Autodesk Fusion 360 part; units mm, degrees
note: some values were not read from the file. Chosen so that the rebuilt part matches the saved one: which bodies a step acts on.
(part 2 of 5)
sketch "スケッチ1 (6)" plane through (0, 0, 0) normal (0, 0, 1) x (1, 0, 0) in component "Stage1_Planet_Gear_C"
  line L0 (-14.59, -15.7128) -> (-14.4842, -14.6573)
  line L1 (-14.4842, -14.6573) -> (-14.5916, -13.8725)
  line L2 (-14.5916, -13.8725) -> (-14.8686, -13.0785)
  line L3 (-14.8686, -13.0785) -> (-15.2722, -12.2874)
  line L4 (-15.2722, -12.2874) -> (-16.2278, -12.2874)
  line L5 (-16.2278, -12.2874) -> (-16.6314, -13.0785)
  line L6 (-16.6314, -13.0785) -> (-16.9084, -13.8725)
  line L7 (-16.9084, -13.8725) -> (-17.0158, -14.6573)
  line L8 (-17.0158, -14.6573) -> (-16.91, -15.7128)
  line L9 (-16.91, -15.7128) -> (-17.7687, -15.8314)
  line L10 (-17.7687, -15.8314) -> (-18.6161, -16.0137)
  line L11 (-18.6161, -16.0137) -> (-18.8777, -14.9856)
  line L12 (-18.8777, -14.9856) -> (-19.2471, -14.2849)
  line L13 (-19.2471, -14.2849) -> (-19.7789, -13.6335)
  line L14 (-19.7789, -13.6335) -> (-20.4287, -13.0281)
  line L15 (-20.4287, -13.0281) -> (-21.3267, -13.355)
  line L16 (-21.3267, -13.355) -> (-21.4354, -14.2364)
  line L17 (-21.4354, -14.2364) -> (-21.4241, -15.0773)
  line L18 (-21.4241, -15.0773) -> (-21.2566, -15.8514)
  line L19 (-21.2566, -15.8514) -> (-20.7962, -16.8071)
  line L20 (-20.7962, -16.8071) -> (-21.5625, -17.2123)
  line L21 (-21.5625, -17.2123) -> (-22.2965, -17.6734)
  line L22 (-22.2965, -17.6734) -> (-22.8939, -16.7967)
  line L23 (-22.8939, -16.7967) -> (-23.4807, -16.2646)
  line L24 (-23.4807, -16.2646) -> (-24.2032, -15.8344)
  line L25 (-24.2032, -15.8344) -> (-25.0209, -15.4878)
  line L26 (-25.0209, -15.4878) -> (-25.753, -16.1021)
  line L27 (-25.753, -16.1021) -> (-25.5536, -16.9675)
  line L28 (-25.5536, -16.9675) -> (-25.2554, -17.7538)
  line L29 (-25.2554, -17.7538) -> (-24.8333, -18.424)
  line L30 (-24.8333, -18.424) -> (-24.0737, -19.1646)
  line L31 (-24.0737, -19.1646) -> (-24.6553, -19.8074)
  line L32 (-24.6553, -19.8074) -> (-25.1873, -20.4917)
  line L33 (-25.1873, -20.4917) -> (-26.0485, -19.8723)
  line L34 (-26.0485, -19.8723) -> (-26.7819, -19.573)
  line L35 (-26.7819, -19.573) -> (-27.608, -19.4158)
  line L36 (-27.608, -19.4158) -> (-28.4949, -19.3698)
  line L37 (-28.4949, -19.3698) -> (-28.9727, -20.1974)
  line L38 (-28.9727, -20.1974) -> (-28.4894, -20.9425)
  line L39 (-28.4894, -20.9425) -> (-27.9402, -21.5793)
  line L40 (-27.9402, -21.5793) -> (-27.3144, -22.0648)
  line L41 (-27.3144, -22.0648) -> (-26.3473, -22.5009)
  line L42 (-26.3473, -22.5009) -> (-26.6739, -23.3038)
  line L43 (-26.6739, -23.3038) -> (-26.9398, -24.1289)
  line L44 (-26.9398, -24.1289) -> (-27.961, -23.8413)
  line L45 (-27.961, -23.8413) -> (-28.7525, -23.8109)
  line L46 (-28.7525, -23.8109) -> (-29.5825, -23.9458)
  line L47 (-29.5825, -23.9458) -> (-30.4316, -24.2058)
  line L48 (-30.4316, -24.2058) -> (-30.5976, -25.147)
  line L49 (-30.5976, -25.147) -> (-29.8886, -25.6818)
  line L50 (-29.8886, -25.6818) -> (-29.1547, -26.0924)
  line L51 (-29.1547, -26.0924) -> (-28.4006, -26.3345)
  line L52 (-28.4006, -26.3345) -> (-27.3427, -26.4136)
  line L53 (-27.3427, -26.4136) -> (-27.375, -27.2798)
  line L54 (-27.375, -27.2798) -> (-27.3427, -28.146)
  line L55 (-27.3427, -28.146) -> (-28.4006, -28.2251)
  line L56 (-28.4006, -28.2251) -> (-29.1547, -28.4672)
  line L57 (-29.1547, -28.4672) -> (-29.8886, -28.8778)
  line L58 (-29.8886, -28.8778) -> (-30.5976, -29.4126)
  line L59 (-30.5976, -29.4126) -> (-30.4316, -30.3538)
  line L60 (-30.4316, -30.3538) -> (-29.5825, -30.6138)
  line L61 (-29.5825, -30.6138) -> (-28.7525, -30.7487)
  line L62 (-28.7525, -30.7487) -> (-27.961, -30.7183)
  line L63 (-27.961, -30.7183) -> (-26.9398, -30.4307)
  line L64 (-26.9398, -30.4307) -> (-26.6739, -31.2558)
  line L65 (-26.6739, -31.2558) -> (-26.3473, -32.0587)
  line L66 (-26.3473, -32.0587) -> (-27.3144, -32.4948)
  line L67 (-27.3144, -32.4948) -> (-27.9402, -32.9803)
  line L68 (-27.9402, -32.9803) -> (-28.4894, -33.6171)
  line L69 (-28.4894, -33.6171) -> (-28.9727, -34.3622)
  line L70 (-28.9727, -34.3622) -> (-28.4949, -35.1898)
  line L71 (-28.4949, -35.1898) -> (-27.608, -35.1438)
  line L72 (-27.608, -35.1438) -> (-26.7819, -34.9866)
  line L73 (-26.7819, -34.9866) -> (-26.0485, -34.6873)
  line L74 (-26.0485, -34.6873) -> (-25.1873, -34.0679)
  line L75 (-25.1873, -34.0679) -> (-24.6553, -34.7522)
  line L76 (-24.6553, -34.7522) -> (-24.0737, -35.395)
  line L77 (-24.0737, -35.395) -> (-24.8333, -36.1356)
  line L78 (-24.8333, -36.1356) -> (-25.2554, -36.8058)
  line L79 (-25.2554, -36.8058) -> (-25.5536, -37.5921)
  line L80 (-25.5536, -37.5921) -> (-25.753, -38.4575)
  line L81 (-25.753, -38.4575) -> (-25.0209, -39.0718)
  line L82 (-25.0209, -39.0718) -> (-24.2032, -38.7252)
  line L83 (-24.2032, -38.7252) -> (-23.4807, -38.295)
  line L84 (-23.4807, -38.295) -> (-22.8939, -37.7629)
  line L85 (-22.8939, -37.7629) -> (-22.2965, -36.8862)
  line L86 (-22.2965, -36.8862) -> (-21.5625, -37.3473)
  line L87 (-21.5625, -37.3473) -> (-20.7962, -37.7525)
  line L88 (-20.7962, -37.7525) -> (-21.2566, -38.7082)
  line L89 (-21.2566, -38.7082) -> (-21.4241, -39.4823)
  line L90 (-21.4241, -39.4823) -> (-21.4354, -40.3232)
  line L91 (-21.4354, -40.3232) -> (-21.3267, -41.2046)
  line L92 (-21.3267, -41.2046) -> (-20.4287, -41.5315)
  line L93 (-20.4287, -41.5315) -> (-19.7789, -40.9261)
  line L94 (-19.7789, -40.9261) -> (-19.2471, -40.2747)
  line L95 (-19.2471, -40.2747) -> (-18.8777, -39.574)
  line L96 (-18.8777, -39.574) -> (-18.6161, -38.5459)
  line L97 (-18.6161, -38.5459) -> (-17.7687, -38.7282)
  line L98 (-17.7687, -38.7282) -> (-16.91, -38.8468)
  line L99 (-16.91, -38.8468) -> (-17.0158, -39.9023)
  line L100 (-17.0158, -39.9023) -> (-16.9084, -40.6871)
  line L101 (-16.9084, -40.6871) -> (-16.6314, -41.4811)
  line L102 (-16.6314, -41.4811) -> (-16.2278, -42.2722)
  line L103 (-16.2278, -42.2722) -> (-15.2722, -42.2722)
  line L104 (-15.2722, -42.2722) -> (-14.8686, -41.4811)
  line L105 (-14.8686, -41.4811) -> (-14.5916, -40.6871)
  line L106 (-14.5916, -40.6871) -> (-14.4842, -39.9023)
  line L107 (-14.4842, -39.9023) -> (-14.59, -38.8468)
  line L108 (-14.59, -38.8468) -> (-13.7313, -38.7282)
  line L109 (-13.7313, -38.7282) -> (-12.8839, -38.5459)
  line L110 (-12.8839, -38.5459) -> (-12.6223, -39.574)
  line L111 (-12.6223, -39.574) -> (-12.2529, -40.2747)
  line L112 (-12.2529, -40.2747) -> (-11.7211, -40.9261)
  line L113 (-11.7211, -40.9261) -> (-11.0713, -41.5315)
  line L114 (-11.0713, -41.5315) -> (-10.1733, -41.2046)
  line L115 (-10.1733, -41.2046) -> (-10.0646, -40.3232)
  line L116 (-10.0646, -40.3232) -> (-10.0759, -39.4823)
  line L117 (-10.0759, -39.4823) -> (-10.2434, -38.7082)
  line L118 (-10.2434, -38.7082) -> (-10.7038, -37.7525)
  line L119 (-10.7038, -37.7525) -> (-9.9375, -37.3473)
  line L120 (-9.9375, -37.3473) -> (-9.2035, -36.8862)
  line L121 (-9.2035, -36.8862) -> (-8.6061, -37.7629)
  line L122 (-8.6061, -37.7629) -> (-8.0193, -38.295)
  line L123 (-8.0193, -38.295) -> (-7.2968, -38.7252)
  line L124 (-7.2968, -38.7252) -> (-6.4791, -39.0718)
  line L125 (-6.4791, -39.0718) -> (-5.747, -38.4575)
  line L126 (-5.747, -38.4575) -> (-5.9464, -37.5921)
  line L127 (-5.9464, -37.5921) -> (-6.2446, -36.8058)
  line L128 (-6.2446, -36.8058) -> (-6.6667, -36.1356)
  line L129 (-6.6667, -36.1356) -> (-7.4263, -35.395)
  line L130 (-7.4263, -35.395) -> (-6.8447, -34.7522)
  line L131 (-6.8447, -34.7522) -> (-6.3127, -34.0679)
  line L132 (-6.3127, -34.0679) -> (-5.4515, -34.6873)
  line L133 (-5.4515, -34.6873) -> (-4.7181, -34.9866)
  line L134 (-4.7181, -34.9866) -> (-3.892, -35.1438)
  line L135 (-3.892, -35.1438) -> (-3.0051, -35.1898)
  line L136 (-3.0051, -35.1898) -> (-2.5273, -34.3622)
  line L137 (-2.5273, -34.3622) -> (-3.0106, -33.6171)
  line L138 (-3.0106, -33.6171) -> (-3.5598, -32.9803)
  line L139 (-3.5598, -32.9803) -> (-4.1856, -32.4948)
  line L140 (-4.1856, -32.4948) -> (-5.1527, -32.0587)
  line L141 (-5.1527, -32.0587) -> (-4.8261, -31.2558)
  line L142 (-4.8261, -31.2558) -> (-4.5602, -30.4307)
  line L143 (-4.5602, -30.4307) -> (-3.539, -30.7183)
  line L144 (-3.539, -30.7183) -> (-2.7475, -30.7487)
  line L145 (-2.7475, -30.7487) -> (-1.9175, -30.6138)
  line L146 (-1.9175, -30.6138) -> (-1.0684, -30.3538)
  line L147 (-1.0684, -30.3538) -> (-0.9024, -29.4126)
  line L148 (-0.9024, -29.4126) -> (-1.6114, -28.8778)
  line L149 (-1.6114, -28.8778) -> (-2.3453, -28.4672)
  line L150 (-2.3453, -28.4672) -> (-3.0994, -28.2251)
  line L151 (-3.0994, -28.2251) -> (-4.1573, -28.146)
  line L152 (-4.1573, -28.146) -> (-4.125, -27.2798)
  line L153 (-4.125, -27.2798) -> (-4.1573, -26.4136)
  line L154 (-4.1573, -26.4136) -> (-3.0994, -26.3345)
  line L155 (-3.0994, -26.3345) -> (-2.3453, -26.0924)
  line L156 (-2.3453, -26.0924) -> (-1.6114, -25.6818)
  line L157 (-1.6114, -25.6818) -> (-0.9024, -25.147)
  line L158 (-0.9024, -25.147) -> (-1.0684, -24.2058)
  line L159 (-1.0684, -24.2058) -> (-1.9175, -23.9458)
  line L160 (-1.9175, -23.9458) -> (-2.7475, -23.8109)
  line L161 (-2.7475, -23.8109) -> (-3.539, -23.8413)
  line L162 (-3.539, -23.8413) -> (-4.5602, -24.1289)
  line L163 (-4.5602, -24.1289) -> (-4.8261, -23.3038)
  line L164 (-4.8261, -23.3038) -> (-5.1527, -22.5009)
  line L165 (-5.1527, -22.5009) -> (-4.1856, -22.0648)
  line L166 (-4.1856, -22.0648) -> (-3.5598, -21.5793)
  line L167 (-3.5598, -21.5793) -> (-3.0106, -20.9425)
  line L168 (-3.0106, -20.9425) -> (-2.5273, -20.1974)
  line L169 (-2.5273, -20.1974) -> (-3.0051, -19.3698)
  line L170 (-3.0051, -19.3698) -> (-3.892, -19.4158)
  line L171 (-3.892, -19.4158) -> (-4.7181, -19.573)
  line L172 (-4.7181, -19.573) -> (-5.4515, -19.8723)
  line L173 (-5.4515, -19.8723) -> (-6.3127, -20.4917)
  line L174 (-6.3127, -20.4917) -> (-6.8447, -19.8074)
  line L175 (-6.8447, -19.8074) -> (-7.4263, -19.1646)
  line L176 (-7.4263, -19.1646) -> (-6.6667, -18.424)
  line L177 (-6.6667, -18.424) -> (-6.2446, -17.7538)
  line L178 (-6.2446, -17.7538) -> (-5.9464, -16.9675)
  line L179 (-5.9464, -16.9675) -> (-5.747, -16.1021)
  line L180 (-5.747, -16.1021) -> (-6.4791, -15.4878)
  line L181 (-6.4791, -15.4878) -> (-7.2968, -15.8344)
  line L182 (-7.2968, -15.8344) -> (-8.0193, -16.2646)
  line L183 (-8.0193, -16.2646) -> (-8.6061, -16.7967)
  line L184 (-8.6061, -16.7967) -> (-9.2035, -17.6734)
  line L185 (-9.2035, -17.6734) -> (-9.9375, -17.2123)
  line L186 (-9.9375, -17.2123) -> (-10.7038, -16.8071)
  line L187 (-10.7038, -16.8071) -> (-10.2434, -15.8514)
  line L188 (-10.2434, -15.8514) -> (-10.0759, -15.0773)
  line L189 (-10.0759, -15.0773) -> (-10.0646, -14.2364)
  line L190 (-10.0646, -14.2364) -> (-10.1733, -13.355)
  line L191 (-10.1733, -13.355) -> (-11.0713, -13.0281)
  line L192 (-11.0713, -13.0281) -> (-11.7211, -13.6335)
  line L193 (-11.7211, -13.6335) -> (-12.2529, -14.2849)
  line L194 (-12.2529, -14.2849) -> (-12.6223, -14.9856)
  line L195 (-12.6223, -14.9856) -> (-12.8839, -16.0137)
  line L196 (-12.8839, -16.0137) -> (-13.7313, -15.8314)
  line L197 (-13.7313, -15.8314) -> (-14.59, -15.7128)
extrude "Stage1_Planet_C_Extrude" add sketch "スケッチ1 (6)" along normal blind 12 from surface at 34 separate body makes body 6 in component "Stage1_Planet_Gear_C"
sketch "スケッチ2 (6)" plane through (0, 0, 0) normal (0, 0, 1) x (1, 0, 0) in component "Stage1_Planet_Gear_C"
  circle A0 centre (-15.75, -27.2798) radius 8
extrude "Stage1_Planet_C_Hub_Lower_Extrude" add sketch "スケッチ2 (6)" along normal blind 3.5 from surface at 30.5 bodies 6 in component "Stage1_Planet_Gear_C"
sketch "スケッチ3 (6)" plane through (0, 0, 0) normal (0, 0, 1) x (1, 0, 0) in component "Stage1_Planet_Gear_C"
  circle A0 centre (-15.75, -27.2798) radius 8
extrude "Stage1_Planet_C_Hub_Upper_Extrude" add sketch "スケッチ3 (6)" along normal blind 3.5 from surface at 46 bodies 6 in component "Stage1_Planet_Gear_C"
sketch "スケッチ4 (6)" plane through (0, 0, 0) normal (0, 0, 1) x (1, 0, 0) in component "Stage1_Planet_Gear_C"
  circle A0 centre (-15.75, -27.2798) radius 4.3
extrude "Stage1_Planet_C_Bore_Cut" cut sketch "スケッチ4 (6)" along normal blind 22 from surface at 29 bodies 6 in component "Stage1_Planet_Gear_C"
sketch "スケッチ1 (7)" plane through (0, 0, 0) normal (0, 0, 1) x (1, 0, 0) in component "Stage1_Internal_Ring_Gear"
  circle A0 centre (0, 0) radius 58
extrude "Stage1_Ring_Extrude" add sketch "スケッチ1 (7)" along normal blind 12 from surface at 34 separate body makes body 7 in component "Stage1_Internal_Ring_Gear"
sketch "スケッチ2 (7)" plane through (0, 0, 0) normal (0, 0, 1) x (1, 0, 0) in component "Stage1_Internal_Ring_Gear"
  circle A0 centre (0, 0) radius 65.5
extrude "Stage1_Ring_Flange_Extrude" add sketch "スケッチ2 (7)" along normal blind 7 from surface at 36.5 bodies 7 in component "Stage1_Internal_Ring_Gear"
sketch "スケッチ3 (7)" plane through (0, 0, 0) normal (0, 0, 1) x (1, 0, 0) in component "Stage1_Internal_Ring_Gear"
  line L0 (46.8321, -2.0047) -> (45.171, -1.2223)
  line L1 (45.171, -1.2223) -> (43.495, -0.6584)
  line L2 (43.495, -0.6584) -> (43.495, 0.6584)
  line L3 (43.495, 0.6584) -> (45.171, 1.2223)
  line L4 (45.171, 1.2223) -> (46.8321, 2.0047)
  line L5 (46.8321, 2.0047) -> (46.8108, 2.4532)
  line L6 (46.8108, 2.4532) -> (46.7851, 2.9016)
  line L7 (46.7851, 2.9016) -> (45.0513, 3.506)
  line L8 (45.0513, 3.506) -> (43.3256, 3.8917)
  line L9 (43.3256, 3.8917) -> (43.1879, 5.2013)
  line L10 (43.1879, 5.2013) -> (44.7957, 5.9373)
  line L11 (44.7957, 5.9373) -> (46.366, 6.889)
  line L12 (46.366, 6.889) -> (46.2979, 7.3329)
  line L13 (46.2979, 7.3329) -> (46.2255, 7.7761)
  line L14 (46.2255, 7.7761) -> (44.438, 8.196)
  line L15 (44.438, 8.196) -> (42.6814, 8.3991)
  line L16 (42.6814, 8.3991) -> (42.4077, 9.6871)
  line L17 (42.4077, 9.6871) -> (43.9297, 10.5872)
  line L18 (43.9297, 10.5872) -> (45.3919, 11.6978)
  line L19 (45.3919, 11.6978) -> (45.2778, 12.1321)
  line L20 (45.2778, 12.1321) -> (45.1595, 12.5653)
  line L21 (45.1595, 12.5653) -> (43.3379, 12.7961)
  line L22 (43.3379, 12.7961) -> (41.5697, 12.8145)
  line L23 (41.5697, 12.8145) -> (41.1628, 14.0669)
  line L24 (41.1628, 14.0669) -> (42.5824, 15.1211)
  line L25 (42.5824, 15.1211) -> (43.9205, 16.3785)
  line L26 (43.9205, 16.3785) -> (43.7616, 16.7985)
  line L27 (43.7616, 16.7985) -> (43.5986, 17.217)
  line L28 (43.5986, 17.217) -> (41.7629, 17.256)
  line L29 (41.7629, 17.256) -> (40.0025, 17.0895)
  line L30 (40.0025, 17.0895) -> (39.4669, 18.2925)
  line L31 (39.4669, 18.2925) -> (40.7686, 19.4893)
  line L32 (40.7686, 19.4893) -> (41.9679, 20.8797)
  line L33 (41.9679, 20.8797) -> (41.7659, 21.2808)
  line L34 (41.7659, 21.2808) -> (41.5601, 21.6799)
  line L35 (41.5601, 21.6799) -> (39.7304, 21.5269)
  line L36 (39.7304, 21.5269) -> (37.997, 21.1773)
  line L37 (37.997, 21.1773) -> (37.3386, 22.3177)
  line L38 (37.3386, 22.3177) -> (38.508, 23.644)
  line L39 (38.508, 23.644) -> (39.5555, 25.1522)
  line L40 (39.5555, 25.1522) -> (39.3127, 25.53)
  line L41 (39.3127, 25.53) -> (39.0663, 25.9054)
  line L42 (39.0663, 25.9054) -> (37.2625, 25.5619)
  line L43 (37.2625, 25.5619) -> (35.5752, 25.0331)
  line L44 (35.5752, 25.0331) -> (34.8012, 26.0984)
  line L45 (34.8012, 26.0984) -> (35.8256, 27.5397)
  line L46 (35.8256, 27.5397) -> (36.7096, 29.1491)
  line L47 (36.7096, 29.1491) -> (36.4287, 29.4994)
  line L48 (36.4287, 29.4994) -> (36.1444, 29.847)
  line L49 (36.1444, 29.847) -> (34.3865, 29.3169)
  line L50 (34.3865, 29.3169) -> (32.7636, 28.6146)
  line L51 (32.7636, 28.6146) -> (31.8825, 29.5931)
  line L52 (31.8825, 29.5931) -> (32.7507, 31.1336)
  line L53 (32.7507, 31.1336) -> (33.4616, 32.8266)
  line L54 (33.4616, 32.8266) -> (33.1456, 33.1456)
  line L55 (33.1456, 33.1456) -> (32.8266, 33.4616)
  line L56 (32.8266, 33.4616) -> (31.1336, 32.7507)
  line L57 (31.1336, 32.7507) -> (29.5931, 31.8825)
  line L58 (29.5931, 31.8825) -> (28.6146, 32.7636)
  line L59 (28.6146, 32.7636) -> (29.3169, 34.3865)
  line L60 (29.3169, 34.3865) -> (29.847, 36.1444)
  line L61 (29.847, 36.1444) -> (29.4994, 36.4287)
  line L62 (29.4994, 36.4287) -> (29.1491, 36.7096)
  line L63 (29.1491, 36.7096) -> (27.5397, 35.8256)
  line L64 (27.5397, 35.8256) -> (26.0984, 34.8012)
  line L65 (26.0984, 34.8012) -> (25.0331, 35.5752)
  line L66 (25.0331, 35.5752) -> (25.5619, 37.2625)
  line L67 (25.5619, 37.2625) -> (25.9054, 39.0663)
  line L68 (25.9054, 39.0663) -> (25.53, 39.3127)
  line L69 (25.53, 39.3127) -> (25.1522, 39.5555)
  line L70 (25.1522, 39.5555) -> (23.644, 38.508)
  line L71 (23.644, 38.508) -> (22.3177, 37.3386)
  line L72 (22.3177, 37.3386) -> (21.1773, 37.997)
  line L73 (21.1773, 37.997) -> (21.5269, 39.7304)
  line L74 (21.5269, 39.7304) -> (21.6799, 41.5601)
  line L75 (21.6799, 41.5601) -> (21.2808, 41.7659)
  line L76 (21.2808, 41.7659) -> (20.8797, 41.9679)
  line L77 (20.8797, 41.9679) -> (19.4893, 40.7686)
  line L78 (19.4893, 40.7686) -> (18.2925, 39.4669)
  line L79 (18.2925, 39.4669) -> (17.0895, 40.0025)
  line L80 (17.0895, 40.0025) -> (17.256, 41.7629)
  line L81 (17.256, 41.7629) -> (17.217, 43.5986)
  line L82 (17.217, 43.5986) -> (16.7985, 43.7616)
  line L83 (16.7985, 43.7616) -> (16.3785, 43.9205)
  line L84 (16.3785, 43.9205) -> (15.1211, 42.5824)
  line L85 (15.1211, 42.5824) -> (14.0669, 41.1628)
  line L86 (14.0669, 41.1628) -> (12.8145, 41.5697)
  line L87 (12.8145, 41.5697) -> (12.7961, 43.3379)
  line L88 (12.7961, 43.3379) -> (12.5653, 45.1595)
  line L89 (12.5653, 45.1595) -> (12.1321, 45.2778)
  line L90 (12.1321, 45.2778) -> (11.6978, 45.3919)
  line L91 (11.6978, 45.3919) -> (10.5872, 43.9297)
  line L92 (10.5872, 43.9297) -> (9.6871, 42.4077)
  line L93 (9.6871, 42.4077) -> (8.3991, 42.6814)
  line L94 (8.3991, 42.6814) -> (8.196, 44.438)
  line L95 (8.196, 44.438) -> (7.7761, 46.2255)
  line L96 (7.7761, 46.2255) -> (7.3329, 46.2979)
  line L97 (7.3329, 46.2979) -> (6.889, 46.366)
  line L98 (6.889, 46.366) -> (5.9373, 44.7957)
  line L99 (5.9373, 44.7957) -> (5.2013, 43.1879)
  line L100 (5.2013, 43.1879) -> (3.8917, 43.3256)
  line L101 (3.8917, 43.3256) -> (3.506, 45.0513)
  line L102 (3.506, 45.0513) -> (2.9016, 46.7851)
  line L103 (2.9016, 46.7851) -> (2.4532, 46.8108)
  line L104 (2.4532, 46.8108) -> (2.0047, 46.8321)
  line L105 (2.0047, 46.8321) -> (1.2223, 45.171)
  line L106 (1.2223, 45.171) -> (0.6584, 43.495)
  line L107 (0.6584, 43.495) -> (-0.6584, 43.495)
  line L108 (-0.6584, 43.495) -> (-1.2223, 45.171)
  line L109 (-1.2223, 45.171) -> (-2.0047, 46.8321)
  line L110 (-2.0047, 46.8321) -> (-2.4532, 46.8108)
  line L111 (-2.4532, 46.8108) -> (-2.9016, 46.7851)
  line L112 (-2.9016, 46.7851) -> (-3.506, 45.0513)
  line L113 (-3.506, 45.0513) -> (-3.8917, 43.3256)
  line L114 (-3.8917, 43.3256) -> (-5.2013, 43.1879)
  line L115 (-5.2013, 43.1879) -> (-5.9373, 44.7957)
  line L116 (-5.9373, 44.7957) -> (-6.889, 46.366)
  line L117 (-6.889, 46.366) -> (-7.3329, 46.2979)
  line L118 (-7.3329, 46.2979) -> (-7.7761, 46.2255)
  line L119 (-7.7761, 46.2255) -> (-8.196, 44.438)
  line L120 (-8.196, 44.438) -> (-8.3991, 42.6814)
  line L121 (-8.3991, 42.6814) -> (-9.6871, 42.4077)
  line L122 (-9.6871, 42.4077) -> (-10.5872, 43.9297)
  line L123 (-10.5872, 43.9297) -> (-11.6978, 45.3919)
  line L124 (-11.6978, 45.3919) -> (-12.1321, 45.2778)
  line L125 (-12.1321, 45.2778) -> (-12.5653, 45.1595)
  line L126 (-12.5653, 45.1595) -> (-12.7961, 43.3379)
  line L127 (-12.7961, 43.3379) -> (-12.8145, 41.5697)
  line L128 (-12.8145, 41.5697) -> (-14.0669, 41.1628)
  line L129 (-14.0669, 41.1628) -> (-15.1211, 42.5824)
  line L130 (-15.1211, 42.5824) -> (-16.3785, 43.9205)
  line L131 (-16.3785, 43.9205) -> (-16.7985, 43.7616)
  line L132 (-16.7985, 43.7616) -> (-17.217, 43.5986)
  line L133 (-17.217, 43.5986) -> (-17.256, 41.7629)
  line L134 (-17.256, 41.7629) -> (-17.0895, 40.0025)
  line L135 (-17.0895, 40.0025) -> (-18.2925, 39.4669)
  line L136 (-18.2925, 39.4669) -> (-19.4893, 40.7686)
  line L137 (-19.4893, 40.7686) -> (-20.8797, 41.9679)
  line L138 (-20.8797, 41.9679) -> (-21.2808, 41.7659)
  line L139 (-21.2808, 41.7659) -> (-21.6799, 41.5601)
  line L140 (-21.6799, 41.5601) -> (-21.5269, 39.7304)
  line L141 (-21.5269, 39.7304) -> (-21.1773, 37.997)
  line L142 (-21.1773, 37.997) -> (-22.3177, 37.3386)
  line L143 (-22.3177, 37.3386) -> (-23.644, 38.508)
  line L144 (-23.644, 38.508) -> (-25.1522, 39.5555)
  line L145 (-25.1522, 39.5555) -> (-25.53, 39.3127)
  line L146 (-25.53, 39.3127) -> (-25.9054, 39.0663)
  line L147 (-25.9054, 39.0663) -> (-25.5619, 37.2625)
  line L148 (-25.5619, 37.2625) -> (-25.0331, 35.5752)
  line L149 (-25.0331, 35.5752) -> (-26.0984, 34.8012)
  line L150 (-26.0984, 34.8012) -> (-27.5397, 35.8256)
  line L151 (-27.5397, 35.8256) -> (-29.1491, 36.7096)
  line L152 (-29.1491, 36.7096) -> (-29.4994, 36.4287)
  line L153 (-29.4994, 36.4287) -> (-29.847, 36.1444)
  line L154 (-29.847, 36.1444) -> (-29.3169, 34.3865)
  line L155 (-29.3169, 34.3865) -> (-28.6146, 32.7636)
  line L156 (-28.6146, 32.7636) -> (-29.5931, 31.8825)
  line L157 (-29.5931, 31.8825) -> (-31.1336, 32.7507)
  line L158 (-31.1336, 32.7507) -> (-32.8266, 33.4616)
  line L159 (-32.8266, 33.4616) -> (-33.1456, 33.1456)
  line L160 (-33.1456, 33.1456) -> (-33.4616, 32.8266)
  line L161 (-33.4616, 32.8266) -> (-32.7507, 31.1336)
  line L162 (-32.7507, 31.1336) -> (-31.8825, 29.5931)
  line L163 (-31.8825, 29.5931) -> (-32.7636, 28.6146)
  line L164 (-32.7636, 28.6146) -> (-34.3865, 29.3169)
  line L165 (-34.3865, 29.3169) -> (-36.1444, 29.847)
  line L166 (-36.1444, 29.847) -> (-36.4287, 29.4994)
  line L167 (-36.4287, 29.4994) -> (-36.7096, 29.1491)
  line L168 (-36.7096, 29.1491) -> (-35.8256, 27.5397)
  line L169 (-35.8256, 27.5397) -> (-34.8012, 26.0984)
  line L170 (-34.8012, 26.0984) -> (-35.5752, 25.0331)
  line L171 (-35.5752, 25.0331) -> (-37.2625, 25.5619)
  line L172 (-37.2625, 25.5619) -> (-39.0663, 25.9054)
  line L173 (-39.0663, 25.9054) -> (-39.3127, 25.53)
  line L174 (-39.3127, 25.53) -> (-39.5555, 25.1522)
  line L175 (-39.5555, 25.1522) -> (-38.508, 23.644)
  line L176 (-38.508, 23.644) -> (-37.3386, 22.3177)
  line L177 (-37.3386, 22.3177) -> (-37.997, 21.1773)
  line L178 (-37.997, 21.1773) -> (-39.7304, 21.5269)
  line L179 (-39.7304, 21.5269) -> (-41.5601, 21.6799)
  line L180 (-41.5601, 21.6799) -> (-41.7659, 21.2808)
  line L181 (-41.7659, 21.2808) -> (-41.9679, 20.8797)
  line L182 (-41.9679, 20.8797) -> (-40.7686, 19.4893)
  line L183 (-40.7686, 19.4893) -> (-39.4669, 18.2925)
  line L184 (-39.4669, 18.2925) -> (-40.0025, 17.0895)
  line L185 (-40.0025, 17.0895) -> (-41.7629, 17.256)
  line L186 (-41.7629, 17.256) -> (-43.5986, 17.217)
  line L187 (-43.5986, 17.217) -> (-43.7616, 16.7985)
  line L188 (-43.7616, 16.7985) -> (-43.9205, 16.3785)
  line L189 (-43.9205, 16.3785) -> (-42.5824, 15.1211)
  line L190 (-42.5824, 15.1211) -> (-41.1628, 14.0669)
  line L191 (-41.1628, 14.0669) -> (-41.5697, 12.8145)
  line L192 (-41.5697, 12.8145) -> (-43.3379, 12.7961)
  line L193 (-43.3379, 12.7961) -> (-45.1595, 12.5653)
  line L194 (-45.1595, 12.5653) -> (-45.2778, 12.1321)
  line L195 (-45.2778, 12.1321) -> (-45.3919, 11.6978)
  line L196 (-45.3919, 11.6978) -> (-43.9297, 10.5872)
  line L197 (-43.9297, 10.5872) -> (-42.4077, 9.6871)
  line L198 (-42.4077, 9.6871) -> (-42.6814, 8.3991)
  line L199 (-42.6814, 8.3991) -> (-44.438, 8.196)
  line L200 (-44.438, 8.196) -> (-46.2255, 7.7761)
  line L201 (-46.2255, 7.7761) -> (-46.2979, 7.3329)
  line L202 (-46.2979, 7.3329) -> (-46.366, 6.889)
  line L203 (-46.366, 6.889) -> (-44.7957, 5.9373)
  line L204 (-44.7957, 5.9373) -> (-43.1879, 5.2013)
  line L205 (-43.1879, 5.2013) -> (-43.3256, 3.8917)
  line L206 (-43.3256, 3.8917) -> (-45.0513, 3.506)
  line L207 (-45.0513, 3.506) -> (-46.7851, 2.9016)
  line L208 (-46.7851, 2.9016) -> (-46.8108, 2.4532)
  line L209 (-46.8108, 2.4532) -> (-46.8321, 2.0047)
  line L210 (-46.8321, 2.0047) -> (-45.171, 1.2223)
  line L211 (-45.171, 1.2223) -> (-43.495, 0.6584)
  line L212 (-43.495, 0.6584) -> (-43.495, -0.6584)
  line L213 (-43.495, -0.6584) -> (-45.171, -1.2223)
  line L214 (-45.171, -1.2223) -> (-46.8321, -2.0047)
  line L215 (-46.8321, -2.0047) -> (-46.8108, -2.4532)
  line L216 (-46.8108, -2.4532) -> (-46.7851, -2.9016)
  line L217 (-46.7851, -2.9016) -> (-45.0513, -3.506)
  line L218 (-45.0513, -3.506) -> (-43.3256, -3.8917)
  line L219 (-43.3256, -3.8917) -> (-43.1879, -5.2013)
  line L220 (-43.1879, -5.2013) -> (-44.7957, -5.9373)
  line L221 (-44.7957, -5.9373) -> (-46.366, -6.889)
  line L222 (-46.366, -6.889) -> (-46.2979, -7.3329)
  line L223 (-46.2979, -7.3329) -> (-46.2255, -7.7761)
  line L224 (-46.2255, -7.7761) -> (-44.438, -8.196)
  line L225 (-44.438, -8.196) -> (-42.6814, -8.3991)
  line L226 (-42.6814, -8.3991) -> (-42.4077, -9.6871)
  line L227 (-42.4077, -9.6871) -> (-43.9297, -10.5872)
  line L228 (-43.9297, -10.5872) -> (-45.3919, -11.6978)
  line L229 (-45.3919, -11.6978) -> (-45.2778, -12.1321)
  line L230 (-45.2778, -12.1321) -> (-45.1595, -12.5653)
  line L231 (-45.1595, -12.5653) -> (-43.3379, -12.7961)
  line L232 (-43.3379, -12.7961) -> (-41.5697, -12.8145)
  line L233 (-41.5697, -12.8145) -> (-41.1628, -14.0669)
  line L234 (-41.1628, -14.0669) -> (-42.5824, -15.1211)
  line L235 (-42.5824, -15.1211) -> (-43.9205, -16.3785)
  line L236 (-43.9205, -16.3785) -> (-43.7616, -16.7985)
  line L237 (-43.7616, -16.7985) -> (-43.5986, -17.217)
  line L238 (-43.5986, -17.217) -> (-41.7629, -17.256)
  line L239 (-41.7629, -17.256) -> (-40.0025, -17.0895)
  line L240 (-40.0025, -17.0895) -> (-39.4669, -18.2925)
  line L241 (-39.4669, -18.2925) -> (-40.7686, -19.4893)
  line L242 (-40.7686, -19.4893) -> (-41.9679, -20.8797)
  line L243 (-41.9679, -20.8797) -> (-41.7659, -21.2808)
  line L244 (-41.7659, -21.2808) -> (-41.5601, -21.6799)
  line L245 (-41.5601, -21.6799) -> (-39.7304, -21.5269)
  line L246 (-39.7304, -21.5269) -> (-37.997, -21.1773)
  line L247 (-37.997, -21.1773) -> (-37.3386, -22.3177)
  line L248 (-37.3386, -22.3177) -> (-38.508, -23.644)
  line L249 (-38.508, -23.644) -> (-39.5555, -25.1522)
  line L250 (-39.5555, -25.1522) -> (-39.3127, -25.53)
  line L251 (-39.3127, -25.53) -> (-39.0663, -25.9054)
  line L252 (-39.0663, -25.9054) -> (-37.2625, -25.5619)
  line L253 (-37.2625, -25.5619) -> (-35.5752, -25.0331)
  line L254 (-35.5752, -25.0331) -> (-34.8012, -26.0984)
  line L255 (-34.8012, -26.0984) -> (-35.8256, -27.5397)
  line L256 (-35.8256, -27.5397) -> (-36.7096, -29.1491)
  line L257 (-36.7096, -29.1491) -> (-36.4287, -29.4994)
  line L258 (-36.4287, -29.4994) -> (-36.1444, -29.847)
  line L259 (-36.1444, -29.847) -> (-34.3865, -29.3169)
  line L260 (-34.3865, -29.3169) -> (-32.7636, -28.6146)
  line L261 (-32.7636, -28.6146) -> (-31.8825, -29.5931)
  line L262 (-31.8825, -29.5931) -> (-32.7507, -31.1336)
  line L263 (-32.7507, -31.1336) -> (-33.4616, -32.8266)
  line L264 (-33.4616, -32.8266) -> (-33.1456, -33.1456)
  line L265 (-33.1456, -33.1456) -> (-32.8266, -33.4616)
  line L266 (-32.8266, -33.4616) -> (-31.1336, -32.7507)
  line L267 (-31.1336, -32.7507) -> (-29.5931, -31.8825)
  line L268 (-29.5931, -31.8825) -> (-28.6146, -32.7636)
  line L269 (-28.6146, -32.7636) -> (-29.3169, -34.3865)
  line L270 (-29.3169, -34.3865) -> (-29.847, -36.1444)
  line L271 (-29.847, -36.1444) -> (-29.4994, -36.4287)
  line L272 (-29.4994, -36.4287) -> (-29.1491, -36.7096)
  line L273 (-29.1491, -36.7096) -> (-27.5397, -35.8256)
  line L274 (-27.5397, -35.8256) -> (-26.0984, -34.8012)
  line L275 (-26.0984, -34.8012) -> (-25.0331, -35.5752)
  line L276 (-25.0331, -35.5752) -> (-25.5619, -37.2625)
  line L277 (-25.5619, -37.2625) -> (-25.9054, -39.0663)
  line L278 (-25.9054, -39.0663) -> (-25.53, -39.3127)
  line L279 (-25.53, -39.3127) -> (-25.1522, -39.5555)
  line L280 (-25.1522, -39.5555) -> (-23.644, -38.508)
  line L281 (-23.644, -38.508) -> (-22.3177, -37.3386)
  line L282 (-22.3177, -37.3386) -> (-21.1773, -37.997)
  line L283 (-21.1773, -37.997) -> (-21.5269, -39.7304)
  line L284 (-21.5269, -39.7304) -> (-21.6799, -41.5601)
  line L285 (-21.6799, -41.5601) -> (-21.2808, -41.7659)
  line L286 (-21.2808, -41.7659) -> (-20.8797, -41.9679)
  line L287 (-20.8797, -41.9679) -> (-19.4893, -40.7686)
  line L288 (-19.4893, -40.7686) -> (-18.2925, -39.4669)
  line L289 (-18.2925, -39.4669) -> (-17.0895, -40.0025)
  line L290 (-17.0895, -40.0025) -> (-17.256, -41.7629)
  line L291 (-17.256, -41.7629) -> (-17.217, -43.5986)
  line L292 (-17.217, -43.5986) -> (-16.7985, -43.7616)
  line L293 (-16.7985, -43.7616) -> (-16.3785, -43.9205)
  line L294 (-16.3785, -43.9205) -> (-15.1211, -42.5824)
  line L295 (-15.1211, -42.5824) -> (-14.0669, -41.1628)
  line L296 (-14.0669, -41.1628) -> (-12.8145, -41.5697)
  line L297 (-12.8145, -41.5697) -> (-12.7961, -43.3379)
  line L298 (-12.7961, -43.3379) -> (-12.5653, -45.1595)
  line L299 (-12.5653, -45.1595) -> (-12.1321, -45.2778)
  line L300 (-12.1321, -45.2778) -> (-11.6978, -45.3919)
  line L301 (-11.6978, -45.3919) -> (-10.5872, -43.9297)
  line L302 (-10.5872, -43.9297) -> (-9.6871, -42.4077)
  line L303 (-9.6871, -42.4077) -> (-8.3991, -42.6814)
  line L304 (-8.3991, -42.6814) -> (-8.196, -44.438)
  line L305 (-8.196, -44.438) -> (-7.7761, -46.2255)
  line L306 (-7.7761, -46.2255) -> (-7.3329, -46.2979)
  line L307 (-7.3329, -46.2979) -> (-6.889, -46.366)
  line L308 (-6.889, -46.366) -> (-5.9373, -44.7957)
  line L309 (-5.9373, -44.7957) -> (-5.2013, -43.1879)
  line L310 (-5.2013, -43.1879) -> (-3.8917, -43.3256)
  line L311 (-3.8917, -43.3256) -> (-3.506, -45.0513)
  line L312 (-3.506, -45.0513) -> (-2.9016, -46.7851)
  line L313 (-2.9016, -46.7851) -> (-2.4532, -46.8108)
  line L314 (-2.4532, -46.8108) -> (-2.0047, -46.8321)
  line L315 (-2.0047, -46.8321) -> (-1.2223, -45.171)
  line L316 (-1.2223, -45.171) -> (-0.6584, -43.495)
  line L317 (-0.6584, -43.495) -> (0.6584, -43.495)
  line L318 (0.6584, -43.495) -> (1.2223, -45.171)
  line L319 (1.2223, -45.171) -> (2.0047, -46.8321)
  line L320 (2.0047, -46.8321) -> (2.4532, -46.8108)
  line L321 (2.4532, -46.8108) -> (2.9016, -46.7851)
  line L322 (2.9016, -46.7851) -> (3.506, -45.0513)
  line L323 (3.506, -45.0513) -> (3.8917, -43.3256)
  line L324 (3.8917, -43.3256) -> (5.2013, -43.1879)
  line L325 (5.2013, -43.1879) -> (5.9373, -44.7957)
  line L326 (5.9373, -44.7957) -> (6.889, -46.366)
  line L327 (6.889, -46.366) -> (7.3329, -46.2979)
  line L328 (7.3329, -46.2979) -> (7.7761, -46.2255)
  line L329 (7.7761, -46.2255) -> (8.196, -44.438)
  line L330 (8.196, -44.438) -> (8.3991, -42.6814)
  line L331 (8.3991, -42.6814) -> (9.6871, -42.4077)
  line L332 (9.6871, -42.4077) -> (10.5872, -43.9297)
  line L333 (10.5872, -43.9297) -> (11.6978, -45.3919)
  line L334 (11.6978, -45.3919) -> (12.1321, -45.2778)
  line L335 (12.1321, -45.2778) -> (12.5653, -45.1595)
  line L336 (12.5653, -45.1595) -> (12.7961, -43.3379)
  line L337 (12.7961, -43.3379) -> (12.8145, -41.5697)
  line L338 (12.8145, -41.5697) -> (14.0669, -41.1628)
  line L339 (14.0669, -41.1628) -> (15.1211, -42.5824)
  line L340 (15.1211, -42.5824) -> (16.3785, -43.9205)
  line L341 (16.3785, -43.9205) -> (16.7985, -43.7616)
  line L342 (16.7985, -43.7616) -> (17.217, -43.5986)
  line L343 (17.217, -43.5986) -> (17.256, -41.7629)
  line L344 (17.256, -41.7629) -> (17.0895, -40.0025)
  line L345 (17.0895, -40.0025) -> (18.2925, -39.4669)
  line L346 (18.2925, -39.4669) -> (19.4893, -40.7686)
  line L347 (19.4893, -40.7686) -> (20.8797, -41.9679)
  line L348 (20.8797, -41.9679) -> (21.2808, -41.7659)
  line L349 (21.2808, -41.7659) -> (21.6799, -41.5601)
  line L350 (21.6799, -41.5601) -> (21.5269, -39.7304)
  line L351 (21.5269, -39.7304) -> (21.1773, -37.997)
  line L352 (21.1773, -37.997) -> (22.3177, -37.3386)
  line L353 (22.3177, -37.3386) -> (23.644, -38.508)
  line L354 (23.644, -38.508) -> (25.1522, -39.5555)
  line L355 (25.1522, -39.5555) -> (25.53, -39.3127)
  line L356 (25.53, -39.3127) -> (25.9054, -39.0663)
  line L357 (25.9054, -39.0663) -> (25.5619, -37.2625)
  line L358 (25.5619, -37.2625) -> (25.0331, -35.5752)
  line L359 (25.0331, -35.5752) -> (26.0984, -34.8012)
  line L360 (26.0984, -34.8012) -> (27.5397, -35.8256)
  line L361 (27.5397, -35.8256) -> (29.1491, -36.7096)
  line L362 (29.1491, -36.7096) -> (29.4994, -36.4287)
  line L363 (29.4994, -36.4287) -> (29.847, -36.1444)
  line L364 (29.847, -36.1444) -> (29.3169, -34.3865)
  line L365 (29.3169, -34.3865) -> (28.6146, -32.7636)
  line L366 (28.6146, -32.7636) -> (29.5931, -31.8825)
  line L367 (29.5931, -31.8825) -> (31.1336, -32.7507)
  line L368 (31.1336, -32.7507) -> (32.8266, -33.4616)
  line L369 (32.8266, -33.4616) -> (33.1456, -33.1456)
  line L370 (33.1456, -33.1456) -> (33.4616, -32.8266)
  line L371 (33.4616, -32.8266) -> (32.7507, -31.1336)
  line L372 (32.7507, -31.1336) -> (31.8825, -29.5931)
  line L373 (31.8825, -29.5931) -> (32.7636, -28.6146)
  line L374 (32.7636, -28.6146) -> (34.3865, -29.3169)
  line L375 (34.3865, -29.3169) -> (36.1444, -29.847)
  line L376 (36.1444, -29.847) -> (36.4287, -29.4994)
  line L377 (36.4287, -29.4994) -> (36.7096, -29.1491)
  line L378 (36.7096, -29.1491) -> (35.8256, -27.5397)
  line L379 (35.8256, -27.5397) -> (34.8012, -26.0984)
  line L380 (34.8012, -26.0984) -> (35.5752, -25.0331)
  line L381 (35.5752, -25.0331) -> (37.2625, -25.5619)
  line L382 (37.2625, -25.5619) -> (39.0663, -25.9054)
  line L383 (39.0663, -25.9054) -> (39.3127, -25.53)
  line L384 (39.3127, -25.53) -> (39.5555, -25.1522)
  line L385 (39.5555, -25.1522) -> (38.508, -23.644)
  line L386 (38.508, -23.644) -> (37.3386, -22.3177)
  line L387 (37.3386, -22.3177) -> (37.997, -21.1773)
  line L388 (37.997, -21.1773) -> (39.7304, -21.5269)
  line L389 (39.7304, -21.5269) -> (41.5601, -21.6799)
  line L390 (41.5601, -21.6799) -> (41.7659, -21.2808)
  line L391 (41.7659, -21.2808) -> (41.9679, -20.8797)
  line L392 (41.9679, -20.8797) -> (40.7686, -19.4893)
  line L393 (40.7686, -19.4893) -> (39.4669, -18.2925)
  line L394 (39.4669, -18.2925) -> (40.0025, -17.0895)
  line L395 (40.0025, -17.0895) -> (41.7629, -17.256)
  line L396 (41.7629, -17.256) -> (43.5986, -17.217)
  line L397 (43.5986, -17.217) -> (43.7616, -16.7985)
  line L398 (43.7616, -16.7985) -> (43.9205, -16.3785)
  line L399 (43.9205, -16.3785) -> (42.5824, -15.1211)
  line L400 (42.5824, -15.1211) -> (41.1628, -14.0669)
  line L401 (41.1628, -14.0669) -> (41.5697, -12.8145)
  line L402 (41.5697, -12.8145) -> (43.3379, -12.7961)
  line L403 (43.3379, -12.7961) -> (45.1595, -12.5653)
  line L404 (45.1595, -12.5653) -> (45.2778, -12.1321)
  line L405 (45.2778, -12.1321) -> (45.3919, -11.6978)
  line L406 (45.3919, -11.6978) -> (43.9297, -10.5872)
  line L407 (43.9297, -10.5872) -> (42.4077, -9.6871)
  line L408 (42.4077, -9.6871) -> (42.6814, -8.3991)
  line L409 (42.6814, -8.3991) -> (44.438, -8.196)
  line L410 (44.438, -8.196) -> (46.2255, -7.7761)
  line L411 (46.2255, -7.7761) -> (46.2979, -7.3329)
  line L412 (46.2979, -7.3329) -> (46.366, -6.889)
  line L413 (46.366, -6.889) -> (44.7957, -5.9373)
  line L414 (44.7957, -5.9373) -> (43.1879, -5.2013)
  line L415 (43.1879, -5.2013) -> (43.3256, -3.8917)
  line L416 (43.3256, -3.8917) -> (45.0513, -3.506)
  line L417 (45.0513, -3.506) -> (46.7851, -2.9016)
  line L418 (46.7851, -2.9016) -> (46.8108, -2.4532)
  line L419 (46.8108, -2.4532) -> (46.8321, -2.0047)
extrude "Stage1_Ring_Teeth_Cut" cut sketch "スケッチ3 (7)" along normal blind 15 from surface at 33 bodies 7 in component "Stage1_Internal_Ring_Gear"
sketch "スケッチ4 (7)" plane through (0, 0, 0) normal (0, 0, 1) x (1, 0, 0) in component "Stage1_Internal_Ring_Gear"
  circle A0 centre (62, 0) radius 3
  circle A1 centre (43.8406, 43.8406) radius 3
  circle A2 centre (0, 62) radius 3
  circle A3 centre (-43.8406, 43.8406) radius 3
  circle A4 centre (-62, 0) radius 3
  circle A5 centre (-43.8406, -43.8406) radius 3
  circle A6 centre (0, -62) radius 3
  circle A7 centre (43.8406, -43.8406) radius 3
extrude "Stage1_Ring_Bolt_Hole_Cut" cut sketch "スケッチ4 (7)" along normal blind 8 from surface at 36 bodies 7 in component "Stage1_Internal_Ring_Gear"
sketch "スケッチ5 (4)" plane through (0, 0, 0) normal (0, 0, 1) x (1, 0, 0) in component "Stage1_Internal_Ring_Gear"
  circle A0 centre (51.1941, 13.7174) radius 3.5
  circle A1 centre (37.4767, 37.4767) radius 3.5
  circle A2 centre (13.7174, 51.1941) radius 3.5
  circle A3 centre (-13.7174, 51.1941) radius 3.5
  circle A4 centre (-37.4767, 37.4767) radius 3.5
  circle A5 centre (-51.1941, 13.7174) radius 3.5
  circle A6 centre (-51.1941, -13.7174) radius 3.5
  circle A7 centre (-37.4767, -37.4767) radius 3.5
  circle A8 centre (-13.7174, -51.1941) radius 3.5
  circle A9 centre (13.7174, -51.1941) radius 3.5
  circle A10 centre (37.4767, -37.4767) radius 3.5
  circle A11 centre (51.1941, -13.7174) radius 3.5
extrude "Stage1_Ring_Lightening_Cut" cut sketch "スケッチ5 (4)" along normal blind 15 from surface at 33 bodies 7 in component "Stage1_Internal_Ring_Gear"
sketch "スケッチ1 (8)" plane through (0, 0, 0) normal (0, 0, 1) x (1, 0, 0) in component "Input_Shaft"
  circle A0 centre (0, 0) radius 10
extrude "Input_Shaft_Main_Extrude" add sketch "スケッチ1 (8)" along normal blind 90 from surface at -44 separate body makes body 8 in component "Input_Shaft"
sketch "スケッチ2 (8)" plane through (0, 0, 0) normal (0, 0, 1) x (1, 0, 0) in component "Input_Shaft"
  circle A0 centre (0, 0) radius 8
extrude "Input_Shaft_Lower_Step_Extrude" add sketch "スケッチ2 (8)" along normal blind 14 from surface at -58 bodies 8 in component "Input_Shaft"
sketch "スケッチ3 (8)" plane through (0, 0, 0) normal (0, 0, 1) x (1, 0, 0) in component "Input_Shaft"
  circle A0 centre (0, 0) radius 13
extrude "Input_Shaft_Bearing_Seat_Extrude" add sketch "スケッチ3 (8)" along normal blind 10 from surface at 15 bodies 8 in component "Input_Shaft"
sketch "スケッチ4 (8)" plane through (0, 0, 0) normal (0, 0, 1) x (1, 0, 0) in component "Input_Shaft"
  line L0 (-3, 8) -> (3, 8)
  line L1 (3, 8) -> (3, 10.5)
  line L2 (3, 10.5) -> (-3, 10.5)
  line L3 (-3, 10.5) -> (-3, 8)
extrude "Input_Shaft_Keyway_Cut" cut sketch "スケッチ4 (8)" along normal blind 14 from surface at 33 bodies 8 in component "Input_Shaft"
sketch "スケッチ5 (5)" plane through (0, 0, 0) normal (0, 0, 1) x (1, 0, 0) in component "Input_Shaft"
  line L0 (-3, 8) -> (3, 8)
  line L1 (3, 8) -> (3, 12.4)
  line L2 (3, 12.4) -> (-3, 12.4)
  line L3 (-3, 12.4) -> (-3, 8)
extrude "Input_Shaft_Key_Extrude" add sketch "スケッチ5 (5)" along normal blind 10 from surface at 35 bodies 8 in component "Input_Shaft"
sketch "スケッチ1 (9)" plane through (0, 0, 0) normal (0, 0, 1) x (1, 0, 0) in component "Input_Handwheel"
  circle A0 centre (0, 0) radius 45
extrude "Handwheel_Rim_Extrude" add sketch "スケッチ1 (9)" along normal blind 10 from surface at -54 separate body makes body 9 in component "Input_Handwheel"
sketch "スケッチ2 (9)" plane through (0, 0, 0) normal (0, 0, 1) x (1, 0, 0) in component "Input_Handwheel"
  circle A0 centre (0, 0) radius 37
extrude "Handwheel_Rim_Bore_Cut" cut sketch "スケッチ2 (9)" along normal blind 12 from surface at -55 bodies 9 in component "Input_Handwheel"
sketch "スケッチ3 (9)" plane through (0, 0, 0) normal (0, 0, 1) x (1, 0, 0) in component "Input_Handwheel"
  circle A0 centre (0, 0) radius 16
extrude "Handwheel_Hub_Extrude" add sketch "スケッチ3 (9)" along normal blind 14 from surface at -56 separate body makes body 10 in component "Input_Handwheel"
sketch "スケッチ4 (9)" plane through (0, 0, 0) normal (0, 0, 1) x (1, 0, 0) in component "Input_Handwheel"
  line L0 (12, -4) -> (40, -4)
  line L1 (40, -4) -> (40, 4)
  line L2 (40, 4) -> (12, 4)
  line L3 (12, 4) -> (12, -4)
  line L4 (7.5124, 10.1766) -> (16.1649, 36.8062)
  line L5 (16.1649, 36.8062) -> (8.5565, 39.2783)
  line L6 (8.5565, 39.2783) -> (-0.096, 12.6487)
  line L7 (-0.096, 12.6487) -> (7.5124, 10.1766)
  line L8 (-7.3571, 10.2895) -> (-30.0095, 26.7475)
  line L9 (-30.0095, 26.7475) -> (-34.7118, 20.2753)
  line L10 (-34.7118, 20.2753) -> (-12.0593, 3.8174)
  line L11 (-12.0593, 3.8174) -> (-7.3571, 10.2895)
  line L12 (-12.0593, -3.8174) -> (-34.7118, -20.2753)
  line L13 (-34.7118, -20.2753) -> (-30.0095, -26.7475)
  line L14 (-30.0095, -26.7475) -> (-7.3571, -10.2895)
  line L15 (-7.3571, -10.2895) -> (-12.0593, -3.8174)
  line L16 (-0.096, -12.6487) -> (8.5565, -39.2783)
  line L17 (8.5565, -39.2783) -> (16.1649, -36.8062)
  line L18 (16.1649, -36.8062) -> (7.5124, -10.1766)
  line L19 (7.5124, -10.1766) -> (-0.096, -12.6487)
extrude "Handwheel_Spoke_Extrude" add sketch "スケッチ4 (9)" along normal blind 6 from surface at -52 bodies 9 10 in component "Input_Handwheel"
sketch "スケッチ5 (6)" plane through (0, 0, 0) normal (0, 0, 1) x (1, 0, 0) in component "Input_Handwheel"
  circle A0 centre (0, 0) radius 8.2
extrude "Handwheel_Bore_Cut" cut sketch "スケッチ5 (6)" along normal blind 18 from surface at -57 bodies 9 in component "Input_Handwheel"
sketch "スケッチ6 (2)" plane through (0, 0, 0) normal (0, 0, 1) x (1, 0, 0) in component "Input_Handwheel"
  circle A0 centre (41, 0) radius 3
  circle A1 centre (28.9914, 28.9914) radius 3
  circle A2 centre (0, 41) radius 3
  circle A3 centre (-28.9914, 28.9914) radius 3
  circle A4 centre (-41, 0) radius 3
  circle A5 centre (-28.9914, -28.9914) radius 3
  circle A6 centre (0, -41) radius 3
  circle A7 centre (28.9914, -28.9914) radius 3
extrude "Handwheel_Grip_Hole_Cut" cut sketch "スケッチ6 (2)" along normal blind 12 from surface at -55 bodies 9 in component "Input_Handwheel"
sketch "スケッチ1 (10)" plane through (0, 0, 0) normal (0, 0, 1) x (1, 0, 0) in component "Stage1_Planet_Carrier"
  circle A0 centre (0, 0) radius 42
extrude "Stage1_Carrier_Lower_Plate_Extrude" add sketch "スケッチ1 (10)" along normal blind 6 from surface at 24 separate body makes body 11 in component "Stage1_Planet_Carrier"
sketch "スケッチ2 (10)" plane through (0, 0, 0) normal (0, 0, 1) x (1, 0, 0) in component "Stage1_Planet_Carrier"
  circle A0 centre (0, 0) radius 20
extrude "Stage1_Carrier_Lower_Bore_Cut" cut sketch "スケッチ2 (10)" along normal blind 8 from surface at 23 bodies 11 in component "Stage1_Planet_Carrier"
sketch "スケッチ3 (10)" plane through (0, 0, 0) normal (0, 0, 1) x (1, 0, 0) in component "Stage1_Planet_Carrier"
  circle A0 centre (15.75, 27.2798) radius 8
  circle A1 centre (-31.5, 0) radius 8
  circle A2 centre (15.75, -27.2798) radius 8
extrude "Stage1_Carrier_Post_Extrude" add sketch "スケッチ3 (10)" along normal blind 20 from surface at 30 bodies 11 in component "Stage1_Planet_Carrier"
sketch "スケッチ4 (10)" plane through (0, 0, 0) normal (0, 0, 1) x (1, 0, 0) in component "Stage1_Planet_Carrier"
  circle A0 centre (0, 0) radius 38
extrude "Stage1_Carrier_Upper_Plate_Extrude" add sketch "スケッチ4 (10)" along normal blind 6 from surface at 50 bodies 11 in component "Stage1_Planet_Carrier"
sketch "スケッチ5 (7)" plane through (0, 0, 0) normal (0, 0, 1) x (1, 0, 0) in component "Stage1_Planet_Carrier"
  circle A0 centre (0, 0) radius 16
extrude "Stage1_Carrier_Hub_Extrude" add sketch "スケッチ5 (7)" along normal blind 6 from surface at 56 bodies 11 in component "Stage1_Planet_Carrier"
sketch "スケッチ6 (3)" plane through (0, 0, 0) normal (0, 0, 1) x (1, 0, 0) in component "Stage1_Planet_Carrier"
  circle A0 centre (32.909, 19) radius 7
  circle A1 centre (0, 38) radius 7
  circle A2 centre (-32.909, 19) radius 7
  circle A3 centre (-32.909, -19) radius 7
  circle A4 centre (0, -38) radius 7
  circle A5 centre (32.909, -19) radius 7
extrude "Stage1_Carrier_Lightening_Cut" cut sketch "スケッチ6 (3)" along normal blind 34 from surface at 23 bodies 11 in component "Stage1_Planet_Carrier"
sketch "スケッチ7 (2)" plane through (0, 0, 0) normal (0, 0, 1) x (1, 0, 0) in component "Stage1_Planet_Carrier"
  circle A0 centre (31.5, 0) radius 4.1
  circle A1 centre (-15.75, 27.2798) radius 4.1
  circle A2 centre (-15.75, -27.2798) radius 4.1
extrude "Stage1_Carrier_Pin_Hole_Cut" cut sketch "スケッチ7 (2)" along normal blind 34 from surface at 23 bodies 11 in component "Stage1_Planet_Carrier"
sketch "スケッチ1 (11)" plane through (0, 0, 0) normal (0, 0, 1) x (1, 0, 0) in component "Intermediate_Shaft"
  circle A0 centre (0, 0) radius 8
extrude "Intermediate_Shaft_Main_Extrude" add sketch "スケッチ1 (11)" along normal blind 33 from surface at 56 separate body makes body 12 in component "Intermediate_Shaft"
sketch "スケッチ2 (11)" plane through (0, 0, 0) normal (0, 0, 1) x (1, 0, 0) in component "Intermediate_Shaft"
  circle A0 centre (0, 0) radius 12
extrude "Intermediate_Shaft_Collar_Extrude" add sketch "スケッチ2 (11)" along normal blind 4 from surface at 64 bodies 12 in component "Intermediate_Shaft"
sketch "スケッチ1 (12)" plane through (0, 0, 0) normal (0, 0, 1) x (1, 0, 0) in component "Stage_Separator_Plate"
  circle A0 centre (0, 0) radius 64
extrude "Stage_Separator_Plate_Extrude" add sketch "スケッチ1 (12)" along normal blind 5 from surface at 58 separate body makes body 13 in component "Stage_Separator_Plate"
sketch "スケッチ2 (12)" plane through (0, 0, 0) normal (0, 0, 1) x (1, 0, 0) in component "Stage_Separator_Plate"
  circle A0 centre (0, 0) radius 24
extrude "Stage_Separator_Center_Bore_Cut" cut sketch "スケッチ2 (12)" along normal blind 7 from surface at 57 bodies 13 in component "Stage_Separator_Plate"
sketch "スケッチ3 (11)" plane through (0, 0, 0) normal (0, 0, 1) x (1, 0, 0) in component "Stage_Separator_Plate"
  circle A0 centre (42, 0) radius 13
  circle A1 centre (21, 36.3731) radius 13
  circle A2 centre (-21, 36.3731) radius 13
  circle A3 centre (-42, 0) radius 13
  circle A4 centre (-21, -36.3731) radius 13
  circle A5 centre (21, -36.3731) radius 13
extrude "Stage_Separator_Window_Cut" cut sketch "スケッチ3 (11)" along normal blind 7 from surface at 57 bodies 13 in component "Stage_Separator_Plate"
sketch "スケッチ4 (11)" plane through (0, 0, 0) normal (0, 0, 1) x (1, 0, 0) in component "Stage_Separator_Plate"
  circle A0 centre (54.5089, 22.5783) radius 3.5
  circle A1 centre (22.5783, 54.5089) radius 3.5
  circle A2 centre (-22.5783, 54.5089) radius 3.5
  circle A3 centre (-54.5089, 22.5783) radius 3.5
  circle A4 centre (-54.5089, -22.5783) radius 3.5
  circle A5 centre (-22.5783, -54.5089) radius 3.5
  circle A6 centre (22.5783, -54.5089) radius 3.5
  circle A7 centre (54.5089, -22.5783) radius 3.5
extrude "Stage_Separator_Bolt_Hole_Cut" cut sketch "スケッチ4 (11)" along normal blind 7 from surface at 57 bodies 13 in component "Stage_Separator_Plate"